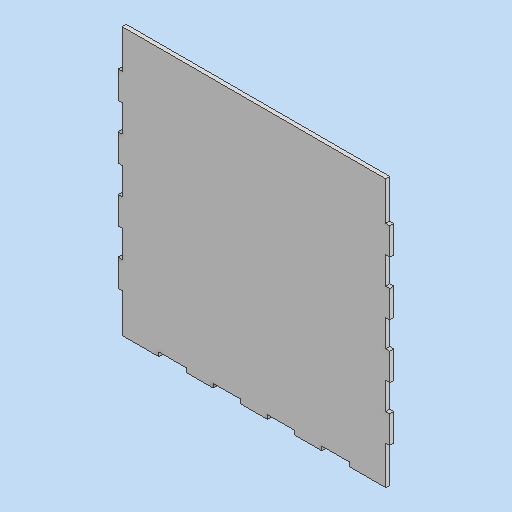
# Autodesk Inventor part: left plate
Saved by Autodesk Inventor 2026 (Build 300175000, 175)
## iProperties
Created: 2026-02-12
Part Number: left plate
Material: Generic
Document SubType Name: Modeling
Designer: mones
Density: 1 g/cm^3
Appearance: Default
Author: mones
Autodesk Inventor part; units mm, degrees
ref_plane "YZ Plane" through (0, 0, 0) normal (1, 0, 0) x (0, 1, 0)
ref_plane "XZ Plane" through (0, 0, 0) normal (0, 1, 0) x (-1, 0, 0)
ref_plane "XY Plane" through (0, 0, 0) normal (0, 0, 1) x (1, 0, 0)
sketch "Sketch1" plane through (0, 0, 0) normal (0, 0, 1) x (1, 0, 0)
  line L0 (-97, 98.5) -> (97, 98.5)
  line L1 (-100, 98.5) -> (100, -98.5) construction
  line L2 (100, 98.5) -> (-100, -98.5) construction
  line L3 (-97, 98.5) -> (-97, 70)
  line L4 (-97, 50) -> (-97, 30)
  line L5 (-97, 10) -> (-97, -10)
  line L6 (-97, -70) -> (-97, -98.5)
  line L7 (-97, 70) -> (-100, 70)
  line L8 (-100, 70) -> (-100, 50)
  line L9 (-100, 30) -> (-100, 10)
  line L10 (-100, -10) -> (-100, -30)
  line L11 (-100, -50) -> (-100, -70)
  line L12 (-100, -70) -> (-97, -70)
  line L13 (-100, -50) -> (-97, -50)
  line L14 (-100, -30) -> (-97, -30)
  line L15 (-100, -10) -> (-97, -10)
  line L16 (-100, 10) -> (-97, 10)
  line L17 (-100, 30) -> (-97, 30)
  line L18 (-100, 50) -> (-97, 50)
  line L19 (97, 98.5) -> (97, 70)
  line L20 (97, 50) -> (97, 30)
  line L21 (97, 10) -> (97, -10)
  line L22 (97, -30) -> (97, -50)
  line L23 (97, -70) -> (97, -98.5)
  line L24 (97, 70) -> (100, 70)
  line L25 (100, 70) -> (100, 50)
  line L26 (100, 30) -> (100, 10)
  line L27 (100, -10) -> (100, -30)
  line L28 (100, -50) -> (100, -70)
  line L29 (100, -70) -> (97, -70)
  line L30 (100, -50) -> (97, -50)
  line L31 (100, -30) -> (97, -30)
  line L32 (100, -10) -> (97, -10)
  line L33 (100, 10) -> (97, 10)
  line L34 (100, 30) -> (97, 30)
  line L35 (100, 50) -> (97, 50)
  line L36 (-100, 50) -> (-100, 70)
  line L37 (-97, 98.5) -> (-97, 70)
  line L38 (-97, 50) -> (-97, 30)
  line L39 (-100, 10) -> (-100, 30)
  line L40 (-97, 10) -> (-97, -10)
  line L41 (-100, -70) -> (-100, -50)
  line L42 (-100, -30) -> (-100, -10)
  line L43 (-97, -30) -> (-97, -50)
  line L44 (-97, -70) -> (-97, -98.5)
  line L45 (100, 50) -> (100, 70)
  line L46 (100, 70) -> (100, 50)
  line L47 (97, 98.5) -> (97, 70)
  line L48 (97, 50) -> (97, 30)
  line L49 (100, 30) -> (100, 10)
  line L50 (100, 10) -> (100, 30)
  line L51 (97, 10) -> (97, -10)
  line L52 (100, -70) -> (100, -50)
  line L53 (100, -30) -> (100, -10)
  line L54 (100, -10) -> (100, -30)
  line L55 (100, -50) -> (100, -70)
  line L56 (97, -30) -> (97, -50)
  line L57 (97, -70) -> (97, -98.5)
  line L58 (-97, -98.5) -> (-70, -98.5)
  line L59 (-50, -98.5) -> (-30, -98.5)
  line L60 (-10, -98.5) -> (10, -98.5)
  line L61 (30, -98.5) -> (50, -98.5)
  line L62 (-97, -98.5) -> (-97, -95.5)
  line L63 (-97, -95.5) -> (97, -95.5) construction
  line L64 (-70, -98.5) -> (-70, -95.5)
  line L65 (-50, -98.5) -> (-50, -95.5)
  line L66 (-30, -98.5) -> (-30, -95.5)
  line L67 (-10, -98.5) -> (-10, -95.5)
  line L68 (10, -98.5) -> (10, -95.5)
  line L69 (30, -98.5) -> (30, -95.5)
  line L70 (50, -98.5) -> (50, -95.5)
  line L71 (70, -98.5) -> (70, -95.5)
  line L72 (97, -98.5) -> (70, -98.5)
  line L73 (50, -95.5) -> (70, -95.5)
  line L74 (50, -98.5) -> (30, -98.5)
  line L75 (10, -95.5) -> (30, -95.5)
  line L76 (10, -98.5) -> (-10, -98.5)
  line L77 (-70, -95.5) -> (-50, -95.5)
  line L78 (-30, -95.5) -> (-10, -95.5)
  line L79 (-30, -98.5) -> (-50, -98.5)
  line L80 (-70, -98.5) -> (-97, -98.5)
  point P0 (0, 0)
  constraints: 160 end point, 58 perpendicular, 28 parallel, 2 midpoint, 2 vertical, 1 horizontal, 1 point on line, 11 other
extrude "Extrusion1" add sketch "Sketch1" along normal blind 3
body "Solid1"
